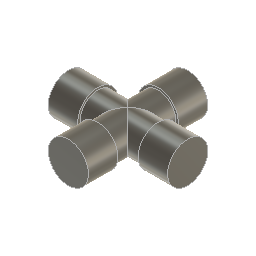
DIY 2DOF Motion Sim Rig (Autodesk Fusion 360 archive; units mm, degrees)
design "U-Joint"
Autodesk Fusion 360 part; units mm, degrees
sketch "Skizze1" plane through (0, 0, 0) normal (0, 1, 0) x (1, 0, 0)
  circle A0 centre (0, 0) radius 15
  dimension "d1" = 30
  constraint coincident A0.centre origin
  measures "d1" diameter of A0
extrude "Extrusion1" add sketch "Skizze1" along normal blind 22 makes body 1
sketch "Skizze2" plane through (0, 22, 0) normal (0, 1, 0) x (-1, 0, 0)
  circle A0 centre (0, 0) radius 15
  circle A1 centre (0, 0) radius 13.25
  dimension "d4" = 26.5
  constraint coincident A0.centre A1.centre
  measures "d4" diameter of A1
extrude "Extrusion2" add sketch "Skizze2" along normal blind 45 contours A1 bodies 1
sketch "Skizze3" plane through (0, 67, 0) normal (0, 1, 0) x (-1, 0, 0)
  circle A0 centre (0, 0) radius 13.25
  circle A1 centre (0, 0) radius 15
  dimension "d7" = 30
  constraint concentric A0 A1
  measures "d7" diameter of A1
extrude "Extrusion3" add sketch "Skizze3" along normal blind 22 contours A0 | A1 bodies 1
move_body "Verschieben1" bodies 1 to x (1, 0, 0) y (0, 1, 0) z (0, 0, 1) at (0, -45, 0)
move_body "Verschieben2" bodies 1 to x (1, 0, 0) y (0, 1, 0) z (0, 0, 1) at (0, 0.5, 0)
sketch "Skizze4" plane through (0, 0, 0) normal (1, 0, 0) x (0, 1, 0)
  circle A0 centre (0, 0) radius 13.25
  dimension "d11" = 26.5
  constraint coincident A0.centre origin
  measures "d11" diameter of A0
extrude "Extrusion4" add sketch "Skizze4" along normal mid plane 71.5 bodies 1
extrude "Extrusion5" cut 1 faces at (35.75, -1.9672, 3.2105) along direction (-1, 0, 0) blind 13.25 on bodies 1 bodies 1
extrude "Extrusion6" cut 1 faces at (-35.75, -1.9672, 3.2105) along direction (1, 0, 0) blind 13.25 on bodies 1 bodies 1
sketch "Skizze5" plane through (22.5, 0, 0) normal (1, 0, 0) x (0, 1, 0)
  circle A0 centre (0, 0) radius 13.25
  circle A1 centre (0, 0) radius 15
  dimension "d18" = 30
  constraint coincident A0.centre A1.centre
  measures "d18" diameter of A1
extrude "Extrusion7" add sketch "Skizze5" along normal blind 22 contours A0 | A1 bodies 1
sketch "Skizze6" plane through (-22.5, 0, 0) normal (-1, 0, 0) x (0, -1, 0)
  circle A0 centre (0, 0) radius 13.25
  circle A1 centre (0, 0) radius 15
  dimension "d21" = 30
  constraint coincident A0.centre A1.centre
  measures "d21" diameter of A1
extrude "Extrusion8" add sketch "Skizze6" along normal blind 22 contours A0 | A1 bodies 1
copy_body "Körper->Berechn1" bodies 1 removing the originals makes body 2 in component "U-Joint"
component "U-Joint" placed x (1, 0, 0) y (0, 1, 0) z (0, 0, 1) at (0, 0, 0)
